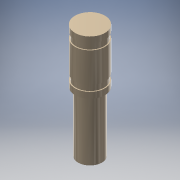
# Autodesk Inventor part: walek popychajacy sprzeglo 01-02
Saved by Autodesk Inventor 2017 (Build 210142000, 142)
## iProperties
Created: 2021-05-23
Part Number: walek popychajacy sprzeglo 01-02
Material: Generic
Document SubType Name: Modeling
Designer: majch
Density: 1 g/cm^3
Appearance: Smooth - Off-White
Mass: 0.297807 g
Surface Area: 3.13562 cm^2
Volume: 0.297807 cm^3
Author: majch
Autodesk Inventor part; units mm, degrees
ref_plane "YZ Plane" through (0, 0, 0) normal (1, 0, 0) x (0, 1, 0)
ref_plane "XZ Plane" through (0, 0, 0) normal (0, 1, 0) x (-1, 0, 0)
ref_plane "XY Plane" through (0, 0, 0) normal (0, 0, 1) x (1, 0, 0)
sketch "Sketch1" plane through (0, 0, 0) normal (0, 1, 0) x (-1, 0, 0)
  line L0 (0, 0) -> (2.5, 0)
  line L1 (2.5, 0) -> (2.5, -1)
  line L2 (2.5, -1) -> (2.35, -1)
  line L3 (2.35, -1) -> (2.35, -2)
  line L4 (2.35, -2) -> (2.5, -2)
  line L5 (2.5, -2) -> (2.5, -7)
  line L6 (2.5, -7) -> (2.35, -7)
  line L7 (2.35, -7) -> (2.35, -8)
  line L8 (2.35, -8) -> (2.5, -8)
  line L9 (2, -19) -> (0, -19)
  line L10 (0, 0) -> (0, -19)
  line L11 (2.5, -8) -> (2.5, -9)
  line L12 (2.5, -9) -> (2, -9)
  line L13 (2, -9) -> (2, -19)
  dimension "d0" = 2.5
  dimension "d1" = 1
  dimension "d2" = 0.15
  dimension "d3" = 1
  dimension "d4" = 5
  dimension "d9" = 2.5
  dimension "d10" = 1
  dimension "d11" = 2
  constraints: 28 end point, 9 perpendicular, 4 vertical, 3 equal length, 1 horizontal
  measures "d0" distance of L0.start L0.end
  measures "d1" distance of L0.end L1.end
  measures "d2" distance of L1.end L2.end
  measures "d3" distance of L2.end L3.end
  measures "d4" distance of L4.end L5.end
  measures "d9" distance between parallel lines of L10 L5
  measures "d10" distance of L8.end L11.end
  measures "d11" distance between parallel lines of L10 L13
revolve "Revolution1" add sketch "Sketch1" angle 360 about axis through (0, 0, 0) along (0, 0, -1)
body "Solid1"
